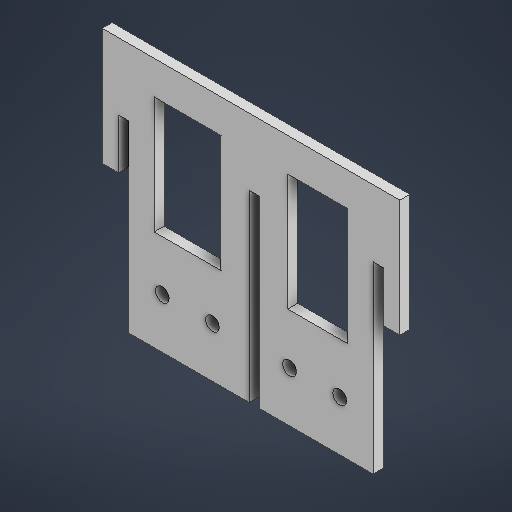
# Autodesk Inventor part: Back_board_large
Saved by Autodesk Inventor 2027 (Build 310192000, 192)
## iProperties
Created: 2026-06-03
Part Number: Back_board_large
Material: Generic
Document SubType Name: Modeling
Designer: alexy
Density: 1 g/cm^3
Appearance: Default
Author: alexy
Autodesk Inventor part; units mm, degrees
ref_plane "YZ Plane" through (0, 0, 0) normal (1, 0, 0) x (0, 1, 0)
ref_plane "XZ Plane" through (0, 0, 0) normal (0, 1, 0) x (-1, 0, 0)
ref_plane "XY Plane" through (0, 0, 0) normal (0, 0, 1) x (1, 0, 0)
sketch "Sketch1" plane through (0, 0, 0) normal (0, 0, 1) x (1, 0, 0)
  line L0 (0, 75) -> (36.05, 75)
  line L1 (36.05, 75) -> (36.05, 0)
  line L2 (36.05, 0) -> (0, 0)
  line L3 (0, 0) -> (0, 75)
  line L4 (36.05, 75) -> (39.05, 75)
  line L5 (39.05, 75) -> (39.05, 55)
  line L6 (39.05, 55) -> (36.05, 55)
  line L7 (36.05, 55) -> (36.05, 75)
  line L8 (39.05, 75) -> (73.1, 75)
  line L9 (73.1, 75) -> (73.1, 0)
  line L10 (73.1, 0) -> (39.05, 0)
  line L11 (39.05, 0) -> (39.05, 75)
  line L12 (0, 75) -> (-3, 75)
  line L13 (-3, 75) -> (-3, 55)
  line L14 (-3, 55) -> (0, 55)
  line L15 (0, 55) -> (0, 75)
  line L16 (73.1, 75) -> (76.1, 75)
  line L17 (76.1, 75) -> (76.1, 55)
  line L18 (76.1, 55) -> (73.1, 55)
  line L19 (73.1, 55) -> (73.1, 75)
  line L20 (76.1, 75) -> (81.1, 75)
  line L21 (81.1, 75) -> (81.1, 40)
  line L22 (81.1, 40) -> (76.1, 40)
  line L23 (76.1, 40) -> (76.1, 75)
  line L24 (-3, 75) -> (-8, 75)
  line L25 (-8, 75) -> (-8, 40)
  line L26 (-8, 40) -> (-3, 40)
  line L27 (-3, 40) -> (-3, 75)
  circle A0 centre (63.1, 15) radius 2.075
  circle A1 centre (10, 15) radius 2.075
  circle A2 centre (25, 15) radius 2.075
  circle A3 centre (48.1, 15) radius 2.075
  point P0 (-3, 55)
  point P1 (0, 55)
  point P2 (36.05, 55)
  point P3 (39.05, 55)
  dimension "d0" = 36.05
  dimension "d1" = 3
  dimension "d2" = 20
  dimension "d3" = 34.05
  dimension "d5" = 75
  dimension "d6" = 3
  dimension "d7" = 3
  dimension "d8" = 5
  dimension "d9" = 35
  dimension "d10" = 5
  dimension "d12" = 4.15
  dimension "d13" = 4.15
  dimension "d14" = 10
  dimension "d15" = 10
  dimension "d16" = 4.15
  dimension "d17" = 4.15
  dimension "d18" = 15
  dimension "d19" = 15
  dimension "d22" = 55
  dimension "d23" = 15
  constraints: 56 end point, 14 parallel, 7 horizontal, 7 perpendicular, 5 horizontal alignment, 4 centre point, 1 coincident, 1 point on line
  measures "d0" distance of L0.start L0.end
  measures "d1" distance of L5.end L6.end
  measures "d2" distance of L0.end L6.end
  measures "d3" distance of L4.end L8.end
  measures "d5" distance of L8.end L9.end
  measures "d6" distance of L0.start L12.end
  measures "d7" distance of L8.end L16.end
  measures "d8" distance of L16.end L20.end
  measures "d9" distance of L20.end L21.end
  measures "d10" distance of L26.end L25.end
  measures "d12" diameter of A0
  measures "d13" diameter of A1
  measures "d14" horizontal distance of point (0, 0) A1.centre
  measures "d15" horizontal distance of L9.end A0.centre
  measures "d16" diameter of A2
  measures "d17" diameter of A3
  measures "d18" distance of A1.centre A2.centre
  measures "d19" distance of A0.centre A3.centre
  measures "d22" distance of point (0, 0) L14.end
  measures "d23" distance from line of L10 A0.centre
extrude "Extrusion1" add sketch "Sketch1" along normal blind 3
sketch "Sketch2" plane through (0, 0, 3) normal (0, 0, 1) x (1, 0, 0)
  line L0 (7.55, 65) -> (27.55, 65)
  line L1 (27.55, 65) -> (27.55, 30)
  line L2 (27.55, 30) -> (7.55, 30)
  line L3 (7.55, 30) -> (7.55, 65)
  line L4 (47.55, 65) -> (65.55, 65)
  line L5 (65.55, 65) -> (65.55, 30)
  line L6 (65.55, 30) -> (47.55, 30)
  line L7 (47.55, 30) -> (47.55, 65)
  line L8 (36.05, 55) -> (39.05, 55) projected
  line L9 (81.1, 75) -> (-8, 75) projected
  point P0 (0, 0)
  point P1 (37.55, 55)
  point P2 (37.55, 55)
  dimension "d24" = 35
  dimension "d25" = 10
  dimension "d26" = 10
  dimension "d27" = 18
  dimension "d28" = 20
  dimension "d29" = 10
  constraints: 16 end point, 4 parallel, 2 horizontal, 2 horizontal alignment, 2 midpoint, 2 perpendicular, 2 point on line
  measures "d24" distance of L4.end L5.end
  measures "d25" horizontal distance of point (37.55, 55) L4.start
  measures "d26" horizontal distance of L0.end point (37.55, 55)
  measures "d27" distance of L4.start L4.end
  measures "d28" distance of L0.start L0.end
  measures "d29" distance between parallel lines of L9 L4
extrude "Extrusion2" cut sketch "Sketch2" against normal blind 3
body "Solid1"
